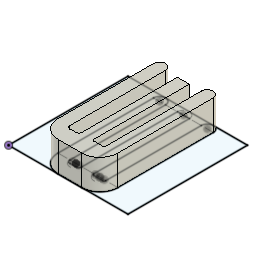
DieShrinkTower v1 (Autodesk Fusion 360 design; units mm, degrees)
Autodesk Fusion 360 part; units mm, degrees
sketch "Sketch1" plane through (0, 0, 0) normal (0, 0, 1) x (1, 0, 0)
  line L0 (0, 0) -> (200, 0)
  line L1 (200, 0) -> (200, 200)
  line L2 (200, 200) -> (0, 200)
  line L3 (0, 200) -> (0, 0)
  line L4 (52.8009, 30) -> (52.8009, 190)
  line L5 (72.8009, 190) -> (72.8009, 30)
  line L6 (112.8009, 190) -> (112.8009, 30)
  line L7 (132.8009, 190) -> (132.8009, 30)
  line L8 (152.8009, 190) -> (152.8009, 30)
  line L9 (52.8009, 190) -> (152.8009, 190) construction
  arc A0 (72.8009, 190) -> (52.8009, 190) centre (62.8009, 190) ccw
  arc A1 (152.8009, 190) -> (132.8009, 190) centre (142.8009, 190) ccw
  line L10 (92.8009, 190) -> (92.8009, 30)
  arc A2 (72.8009, 30) -> (92.8009, 30) centre (82.8009, 30) ccw construction
  arc A3 (112.8009, 30) -> (132.8009, 30) centre (122.8009, 30) ccw construction
  arc A4 (112.8009, 190) -> (92.8009, 190) centre (102.8009, 190) ccw construction
  arc A5 (52.8009, 30) -> (82.8009, 0) centre (82.8009, 30) ccw
  line L11 (92.8009, 190) -> (112.8009, 190)
  arc A6 (72.8009, 30) -> (77.8009, 25) centre (77.8009, 30) ccw
  arc A7 (87.8009, 25) -> (92.8009, 30) centre (87.8009, 30) ccw
  arc A8 (112.8009, 30) -> (115.3009, 27.5) centre (115.3009, 30) ccw
  arc A9 (130.3009, 27.5) -> (132.8009, 30) centre (130.3009, 30) ccw
  line L12 (77.8009, 25) -> (87.8009, 25)
  line L13 (115.3009, 27.5) -> (130.3009, 27.5)
  line L14 (82.8009, 0) -> (122.8009, 0)
  line L15 (52.8009, 30) -> (152.8009, 30) construction
  arc A10 (122.8009, 0) -> (152.8009, 30) centre (122.8009, 30) ccw
  dimension "d1" = 200
  dimension "d2" = 200
  dimension "d3" = 20
  dimension "d4" = 5
  dimension "d5" = 2.5
  dimension "d6" = 62.8009
  constraint horizontal L0
  constraint vertical L1
  constraint horizontal L2
  constraint vertical L3
  constraint coincident L0.start L3.end
  constraint perpendicular L2 L5
  constraint vertical L6
  constraint perpendicular L2 L7
  constraint perpendicular L2 L8
  constraint vertical L4
  constraint perpendicular L8 L9
  constraint coincident L5.start L9
  constraint coincident L6.start L9
  constraint coincident L7.start L9
  constraint coincident L8.start L9.end
  constraint tangent L4 A0
  constraint tangent L7 A1
  constraint coincident L9 L10.start
  constraint perpendicular L9 L10
  constraint tangent L5 A2
  constraint tangent L10 A2
  constraint tangent L6 A3
  constraint tangent L7 A3
  constraint tangent L10 A4
  constraint equal A0 A4
  constraint equal A1 A4
  constraint equal A1 A3
  constraint equal A2 A3
  constraint tangent L2 A0
  constraint coincident A2.centre A5.centre
  constraint tangent L4 A5
  constraint horizontal L12
  constraint horizontal L13
  constraint equal A6 A7
  constraint equal A8 A9
  constraint tangent A6 L12
  constraint tangent A7 L12
  constraint tangent A8 L13
  constraint tangent A9 L13
  constraint tangent L10 A7
  constraint tangent L5 A6
  constraint tangent L6 A8
  constraint horizontal L14
  constraint tangent A5 L14
  constraint horizontal L15
  constraint tangent L8 A10
  constraint tangent L14 A10
  constraint coincident L0 A5.end
  constraint coincident L7.end L15
  measures "d1" distance of L0.start L0.end
  measures "d2" distance of L0.start L2.end
  measures "d3" distance of L4 L5
  measures "d4" radius of A6
  measures "d5" radius of A8
  measures "d6" distance of L3 A0.centre
extrude "Extrude2" add sketch "Sketch1" along normal blind 50 contours L0 L4 L5 L6 L7 L8 A0 A1 L10 A5 L11 A6 A7 A8 A9 L12 L13 L14 A10
